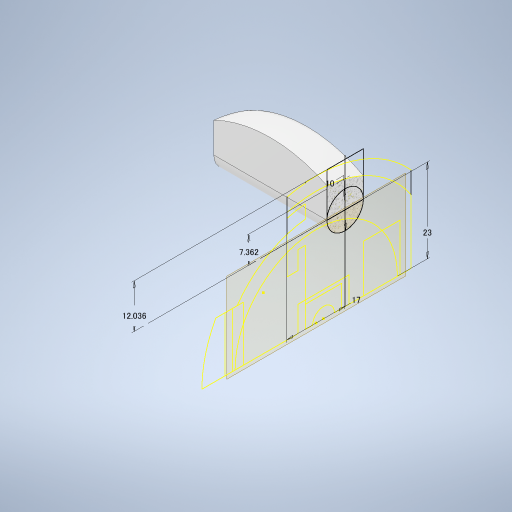
# Autodesk Inventor part: tail11-1
Saved by Autodesk Inventor 2023 (Build 270158000, 158)
## iProperties
Created: 2022-10-08
Part Number: tail11-1
Material: ABS プラスチック
Document SubType Name: Modeling
Designer: ellie
Density: 1.06 g/cm^3
Appearance: 積雪
Author: ellie
Autodesk Inventor part; units mm, degrees
sketch "スケッチ1" plane through (0, 0, 0) normal (0, 1, 0) x (-1, 0, 0)
  circle A0 centre (0, 0) radius 35
  line L0 (0, 0) -> (0, -35)
  line L1 (0, 0) -> (0, 35)
  dimension "d0" = 70
  constraints: 4 end point, 2 point on circle, 2 vertical, 1 centre point, 1 coincident
  measures "d0" diameter of A0
revolve "回転1" add sketch "スケッチ1" angle 180 about axis through (0, 0, 0) along (0, 0, 1) picked at (-2.5961, -23.0408) contours L1 L0 A0
sketch "スケッチ5" plane through (0, 0, 0) normal (0, -1, 0) x (1, 0, 0)
  line L0 (-20, -23) -> (20, -23)
  line L1 (20, -23) -> (20, -13)
  line L2 (20, -13) -> (-20, -13)
  line L3 (-20, -13) -> (-20, -23)
  line L4 (-20, -15) -> (-20, -13)
  line L5 (0, 25) -> (-17, 25)
  line L6 (-17, 25) -> (-17, 23)
  line L7 (-17, 23) -> (0, 23)
  line L8 (0, 23) -> (0, 25)
  line L9 (0, 20) -> (-20, 20)
  line L10 (-20, 20) -> (-20, 19)
  line L11 (-20, 19) -> (0, 19)
  line L12 (0, 19) -> (0, 20)
  line L13 (0, 13) -> (-21, 13)
  line L14 (-21, 13) -> (-21, 11)
  line L15 (-21, 11) -> (0, 11)
  line L16 (0, 11) -> (0, 13)
  line L17 (0, 5) -> (-23, 5)
  line L18 (-23, 5) -> (-23, 3)
  line L19 (-23, 3) -> (0, 3)
  line L20 (0, 3) -> (0, 5)
  circle A0 centre (0, 0) radius 35 projected
  circle A1 centre (0, 0) radius 35 projected
  line L21 (0, 35) -> (0, -35)
  line L22 (35, 0) -> (-35, 0)
  line L23 (-32, 3) -> (-23, 3)
  line L24 (-23, 3) -> (-23, -7)
  line L25 (-23, -7) -> (-32, -7)
  line L26 (-32, -7) -> (-32, 3)
  line L27 (-23, -8.0262) -> (-23, 3)
  line L28 (-27, 22.2711) -> (-27, -22.2711)
  line L29 (-15.5, 25) -> (0, 25)
  line L30 (0, 25) -> (0, 35)
  line L31 (0, 35) -> (-15.5, 35)
  line L32 (-15.5, 35) -> (-15.5, 25)
  line L33 (-15.5, 23) -> (0, 23)
  line L34 (0, 23) -> (0, 20)
  line L35 (0, 20) -> (-15.5, 20)
  line L36 (-15.5, 20) -> (-15.5, 23)
  line L37 (-19, 13) -> (0, 13)
  line L38 (0, 13) -> (0, 19)
  line L39 (0, 19) -> (-19, 19)
  line L40 (-19, 19) -> (-19, 13)
  line L41 (-19, 11) -> (0, 11)
  line L42 (0, 11) -> (0, 5)
  line L43 (0, 5) -> (-19, 5)
  line L44 (-19, 5) -> (-19, 11)
  line L45 (-23, -2) -> (-39.6865, -2)
  line L46 (-23, -2) -> (-7.8337, -2)
  line L47 (-8, 3) -> (-23, 3)
  line L48 (-23, 3) -> (-23, -7)
  line L49 (-23, -7) -> (-8, -7)
  line L50 (-8, -7) -> (-8, 3)
  line L51 (-8, 3) -> (-23, -7) construction
  line L52 (-23, 3) -> (-8, -7) construction
  line L53 (-23, 5) -> (-33, 5)
  line L54 (-33, 5) -> (-33, -9)
  line L55 (-33, -9) -> (-23, -9)
  line L56 (-23, -9) -> (-23, 5)
  line L57 (-23, 5) -> (-33, -9) construction
  line L58 (-33, 5) -> (-23, -9) construction
  line L59 (-8, 3) -> (-1, 3)
  line L60 (-1, 3) -> (-1, -7)
  line L61 (-1, -7) -> (-8, -7)
  line L62 (-8, -7) -> (-8, 3)
  line L63 (-8, 3) -> (-1, -7) construction
  line L64 (-1, 3) -> (-8, -7) construction
  line L65 (-23, 3) -> (-27, 3)
  line L66 (-23, -7) -> (-27, -7)
  line L67 (-23, 5) -> (-27, 5)
  line L68 (-23, -9) -> (-27, -9)
  line L69 (23.4307, -26) -> (-23.4307, -26)
  line L70 (-8, 3) -> (-6.8, 3)
  line L71 (-6.8, 3) -> (-6.8, -7)
  line L72 (-6.8, -7) -> (-8, -7)
  line L73 (-8, -7) -> (-8, 3)
  line L74 (-3, 5) -> (0, 5)
  line L75 (0, 20) -> (-4, 20)
  line L76 (-4, 19) -> (0, 19)
  line L77 (0, 19) -> (0, 20)
  line L78 (-6, 5) -> (-1, 5)
  line L79 (-1, 3) -> (-6, 3)
  point P0 (0, -23)
  point P1 (0, -13)
  point P2 (0, 24)
  point P3 (0, 19.5)
  point P4 (0, 12)
  point P5 (0, 4)
  point P6 (-20, -18)
  point P7 (-27, -0.5262)
  point P8 (-27, -7)
  point P9 (-15.5, 21.5)
  point P10 (-15.5, 31.3807)
  point P11 (0, 25)
  point P12 (0, 23)
  point P13 (0, 11)
  point P14 (0, 13)
  point P15 (-27, 0)
  point P16 (-32, 0)
  point P17 (-23, 0)
  point P18 (-15.5, -2)
  point P19 (-28, -2)
  point P20 (-4.5, -2)
  point P21 (-8, 3)
  point P22 (-27, 0.5)
  point P23 (-28, 0.4738)
  point P24 (-28, -11.5262)
  point P25 (-27, -11.5)
  point P26 (-23, -7)
  point P27 (-23, -7)
  point P28 (-23, -7)
  point P29 (-8, 0)
  point P30 (-1, 0)
  point P31 (0, 19)
  point P32 (0, 20)
  point P33 (-27, -9)
  point P34 (-27, 5)
  dimension "d12" = 40
  dimension "d13" = 10
  dimension "d23" = 17
  dimension "d24" = 2
  dimension "d27" = 20
  dimension "d28" = 1
  dimension "d30" = 21
  dimension "d31" = 2
  dimension "d33" = 2
  dimension "d88" = 0
  dimension "d89" = 0
  dimension "d90" = 12
  dimension "d92" = 20
  dimension "d93" = 10
  dimension "d97" = 9
  dimension "d98" = 10
  dimension "d113" = 27
  dimension "d122" = 15.5
  dimension "d123" = 35
  dimension "d124" = 3
  dimension "d125" = 15.5
  dimension "d126" = 6
  dimension "d127" = 6
  dimension "d128" = 19
  dimension "d129" = 19
  dimension "d147" = 10
  dimension "d149" = 8
  dimension "d151" = 15
  dimension "d161" = 14
  dimension "d162" = 10
  dimension "d164" = 10
  dimension "d165" = 7
  dimension "d170" = 26
  dimension "d175" = 1.2
  dimension "d207" = 0
  constraints: 158 end point, 31 parallel, 20 horizontal, 17 perpendicular, 16 point on line, 15 midpoint, 10 collinear, 1 vertical, 20 other
  measures "d12" distance of L2.end L1.end
  measures "d13" distance of L1.end L0.end
  measures "d23" distance of L7.end L6.end
  measures "d24" distance of L6.end L5.end
  measures "d27" distance of L11.end L10.end
  measures "d28" distance of L10.end L9.end
  measures "d30" distance of L15.end L14.end
  measures "d31" distance of L14.end L13.end
  measures "d33" distance of L18.end L17.end
  measures "d89" distance from line of point (0, 0) L22
  measures "d90" distance from line of L0 point (0, -35)
  measures "d92" distance of the line from the sketch origin of L3
  measures "d93" distance from line of L5 point (0, 35)
  measures "d97" distance of L24.end L25.end
  measures "d98" distance of L23.end L24.end
  measures "d113" distance of the line from the sketch origin of L28
  measures "d122" distance of the line from the sketch origin of L32
  measures "d123" distance between parallel lines of L31 L22
  measures "d124" distance of L33.end L34.end
  measures "d126" distance of L38.end L37.end
  measures "d127" distance of L41.end L42.end
  measures "d128" distance of the line from the sketch origin of L44
  measures "d129" distance of the line from the sketch origin of L40
  measures "d147" distance of L48.end L47.end
  measures "d149" distance of the line from the sketch origin of L50
  measures "d151" distance between parallel lines of L50 L24
  measures "d161" distance between parallel lines of L55 L53
  measures "d162" distance between parallel lines of L48 L54
  measures "d164" distance between parallel lines of L61 L59
  measures "d165" distance between parallel lines of L50 L60
  measures "d170" distance between parallel lines of L69 L22
  measures "d175" distance of L71.end L72.end
  measures "d207" distance between parallel lines of L47 L19
extrude "GNSボード" cut sketch "スケッチ5" against normal blind 16 contours L8 L7 L6 L5
extrude "GNSボード止めるよう" cut sketch "スケッチ5" against normal blind 15 contours L21 L5 L32 A0 | L21 L9 L36 L7
extrude "アルミ板１" cut sketch "スケッチ5" against normal blind 20 contours L11 L10 L9 L12
extrude "メイン基板" cut sketch "スケッチ5" against normal blind 21 contours L15 L14 L13 L16
extrude "メイン止めるよう" cut sketch "スケッチ5" against normal blind 15 contours L17 L44 L15 L21 | L13 L40 L11 L21
extrude "アルミ板２" cut sketch "スケッチ5" against normal blind 20 contours L19 L18 L17 L20
extrude "電池ボックス入れ" cut sketch "スケッチ5" against normal blind 13 contours L3 L2 L21 L0 | L21 L2 L1 L0
extrude "side ut" cut sketch "スケッチ5" against normal blind 100 contours A0 L45 L54 L55 L28 | A0 L22 L54 L45 | L55 L54 L45 L26 L25 L28 | A0 L28 L53 L54 L22 | L54 L22 L26 L45 | L25 L26 L45 L28 | L54 L53 L28 L23 L26 L22 | L26 L22 L28 L45 | L22 L26 L23 L28
extrude "motor case" add sketch "スケッチ5" against normal blind 7 contours L55 L54 L45 L26 L25 L28 | L28 L25 L27 L56 L55 | L50 L46 L24 L22 | L22 L24 L19 L50 | L54 L22 L26 L45 | L28 L45 L24 L25 | L25 L26 L45 L28 | L24 L45 L28 L22 | L22 L28 L23 L24 | L50 L49 L24 L46 | L54 L53 L28 L23 L26 L22 | L26 L22 L28 L45 | L53 L18 L23 L28 | L22 L26 L23 L28
extrude "bottom cut" cut sketch "スケッチ5" against normal blind 90 contours L69 A0 L21 | L21 A0 L69
extrude "motor" cut sketch "スケッチ5" against normal blind 6 contours L60 L61 L71 L22 | L22 L71 L19 L60 | L71 L61 L50 L22 | L22 L50 L19 L71 | L50 L46 L24 L22 | L22 L24 L19 L50 | L28 L45 L24 L25 | L25 L26 L45 L28 | L24 L45 L28 L22 | L22 L28 L23 L24 | L50 L49 L24 L46 | L26 L22 L28 L45 | L22 L26 L23 L28
extrude "motor block" add sketch "スケッチ5" against normal blind 10 contours L71 L61 L50 L22 | L22 L50 L19 L71
sketch "スケッチ27" plane through (-33, 0, -9) normal (-1, 0, 0) x (0, 0, 1)
  line L0 (14, 0) -> (0, 0) projected
  circle A0 centre (7, 0) radius 3
  point P0 (9, 0)
  dimension "d198" = 6
  constraints: 1 centre point, 1 midpoint
  measures "d198" diameter of A0
extrude "moter shaft" cut sketch "スケッチ27" against normal blind 27
mirror "ミラー13" about plane through (0, 0, 0) normal (1, 0, 0) of "メイン止めるよう", "メイン基板", "アルミ板１", "GNSボード止めるよう", "GNSボード", "アルミ板２", "motor", "motor case", "moter shaft", "電池ボックス入れ", "side ut", "motor block"
ref_plane "作業平面5" through (-17, 17.5, 23) normal (0, -1, 0) x (1, 0, 0)
ref_plane "作業平面6" through (20, 13, -13) normal (0, 0, -1) x (1, 0, 0)
ref_plane "作業平面7" through (27, 11.5, 5) normal (0, -1, 0) x (1, 0, 0)
sketch "スケッチ41" plane through (-17, 0, 23) normal (0, -1, 0) x (1, 0, 0)
  line L0 (-16, -22) -> (-15, -22) projected
  line L1 (-15, -22) -> (-15, -20) projected
  line L2 (-15, -20) -> (-6, -20) projected
  line L3 (-6, -20) -> (-6, -18) projected
  line L4 (-6, -18) -> (-2, -18) projected
  line L5 (-2, -18) -> (-2, -12) projected
  line L6 (-2, -12) -> (-4, -12) projected
  line L7 (-4, -12) -> (-4, -10) projected
  line L8 (-4, -10) -> (-2, -10) projected
  line L9 (-2, -10) -> (-2, -4) projected
  line L10 (-2, -4) -> (-3, -4) projected
  line L11 (-3, -4) -> (-3, -3) projected
  line L12 (-3, -3) -> (1.5, -3) projected
  line L13 (1.5, -3) -> (1.5, 0) projected
  line L14 (1.5, 0) -> (0, 0) projected
  line L15 (0, 0) -> (0, 2) projected
  line L16 (0, 2) -> (1.5, 2) projected
  line L17 (1.5, 2) -> (1.5, 8.3807) projected
  arc A0 (1.5, 8.3807) -> (-10, -0.7289) centre (17, -23) ccw projected
  line L18 (-10, -0.7289) -> (-10, -18) projected
  line L19 (-10, -18) -> (-16, -18) projected
  line L20 (-16, -18) -> (-16, -22) projected
  line L21 (-2, -18) -> (-2, -12) projected
  line L22 (-4, -10) -> (-4, -12) projected
  line L23 (0, 2) -> (0, 0) projected
  circle A1 centre (-4, 0.5) radius 2.4
  dimension "d252" = 4.8
  dimension "d253" = 4
  dimension "d254" = 3.5
  constraints: 1 centre point
  measures "d252" diameter of A1
  measures "d253" distance from line of A1.centre L15
  measures "d254" distance from line of A1.centre L12
extrude "top lock 10mm" cut sketch "スケッチ41" against normal blind 3 contours A1
mirror "ミラー15" about plane through (0, 0, 0) normal (1, 0, 0) of "top lock 10mm"
sketch "スケッチ42" plane through (-33, 0, -9) normal (0, -1, 0) x (1, 0, 0)
  circle A0 centre (9.5, -8) radius 2.4
  line L0 (13, -14) -> (13, -4) projected
  line L1 (32, 2) -> (1, 2) projected
  point P0 (33, 9)
  point P1 (10, 2)
  dimension "d257" = 3.5
  dimension "d258" = 4.8
  dimension "d259" = 10
  constraints: 1 centre point
  measures "d257" distance from line of A0.centre L0
  measures "d258" diameter of A0
  measures "d259" distance from line of A0.centre L1
extrude "bottom lock" cut sketch "スケッチ42" against normal blind 3
mirror "ミラー16" about plane through (0, 0, 0) normal (1, 0, 0) of "bottom lock"
ref_plane "作業平面8" through (-17, 15, 23) normal (0, -1, 0) x (1, 0, 0)
sketch "スケッチ45" plane through (-17, 15, 23) normal (0, -1, 0) x (1, 0, 0)
  circle A0 centre (-4, 0.5) radius 2.4 projected
  line L0 (-16, -22) -> (-15, -22) projected
  line L1 (-15, -22) -> (-15, -20) projected
  line L2 (-15, -20) -> (-6, -20) projected
  line L3 (-6, -20) -> (-6, -18) projected
  line L4 (-6, -18) -> (-2, -18) projected
  line L5 (-2, -18) -> (-2, -12) projected
  line L6 (-2, -12) -> (-4, -12) projected
  line L7 (-4, -12) -> (-4, -10) projected
  line L8 (-4, -10) -> (-2, -10) projected
  line L9 (-2, -10) -> (-2, -4) projected
  line L10 (-2, -4) -> (-3, -4) projected
  line L11 (-3, -4) -> (-3, -3) projected
  line L12 (-3, -3) -> (1.5, -3) projected
  line L13 (1.5, -3) -> (1.5, 0) projected
  line L14 (1.5, 0) -> (0, 0) projected
  line L15 (0, 0) -> (0, 2) projected
  line L16 (0, 2) -> (1.5, 2) projected
  line L17 (1.5, 2) -> (1.5, 8.3807) projected
  arc A1 (1.5, 8.3807) -> (-10, -0.7289) centre (17, -23) ccw projected
  line L18 (-10, -0.7289) -> (-10, -18) projected
  line L19 (-10, -18) -> (-16, -18) projected
  line L20 (-16, -18) -> (-16, -22) projected
  arc A2 (32.5, 4.5636) -> (1.5, 4.5636) centre (17, -23) ccw projected
  line L21 (1.5, 2) -> (1.5, 4.5636) projected
  line L22 (32.5, 2) -> (1.5, 2) projected
  line L23 (32.5, 2) -> (32.5, 4.5636) projected
  circle A3 centre (38, 0.5) radius 2.4 projected
  line L24 (49, -22) -> (50, -22) projected
  line L25 (50, -18) -> (50, -22) projected
  line L26 (44, -18) -> (50, -18) projected
  line L27 (44, -18) -> (44, -0.7289) projected
  arc A4 (44, -0.7289) -> (32.5, 8.3807) centre (17, -23) ccw projected
  line L28 (32.5, 8.3807) -> (32.5, 2) projected
  line L29 (32.5, 2) -> (34, 2) projected
  line L30 (34, 2) -> (34, 0) projected
  line L31 (34, 0) -> (32.5, 0) projected
  line L32 (32.5, 0) -> (32.5, -3) projected
  line L33 (32.5, -3) -> (37, -3) projected
  line L34 (37, -3) -> (37, -4) projected
  line L35 (37, -4) -> (36, -4) projected
  line L36 (36, -4) -> (36, -10) projected
  line L37 (36, -10) -> (38, -10) projected
  line L38 (38, -10) -> (38, -12) projected
  line L39 (38, -12) -> (36, -12) projected
  line L40 (36, -12) -> (36, -18) projected
  line L41 (36, -18) -> (40, -18) projected
  line L42 (40, -18) -> (40, -20) projected
  line L43 (40, -20) -> (49, -20) projected
  line L44 (49, -20) -> (49, -22) projected
  circle A5 centre (38, 0.5) radius 2.4 projected
  circle A6 centre (-4, 0.5) radius 2.4 projected
  line L45 (34, 0) -> (0, 0) projected
  line L46 (34, 0) -> (34, 2) projected
  line L47 (34, 2) -> (0, 2) projected
  line L48 (0, 0) -> (0, 2) projected
  line L49 (32.5, -3) -> (1.5, -3) projected
  line L50 (32.5, -3) -> (32.5, 0) projected
  line L51 (1.5, 0) -> (32.5, 0) projected
  line L52 (1.5, -3) -> (1.5, 0) projected
  line L53 (-2, -4) -> (36, -4) projected
  circle A7 centre (38, 0.5) radius 2.4 projected
  line L54 (36, -10) -> (-2, -10) projected
  line L55 (36, -10) -> (36, -4) projected
  line L56 (-2, -4) -> (36, -4) projected
  line L57 (-2, -10) -> (-2, -4) projected
  line L58 (-2, -12) -> (36, -12) projected
  line L59 (36, -18) -> (-2, -18) projected
  line L60 (36, -18) -> (36, -12) projected
  line L61 (-2, -12) -> (36, -12) projected
  line L62 (-2, -18) -> (-2, -12) projected
  line L63 (40, -20) -> (-6, -20) projected
  line L64 (40, -20) -> (40, -18) projected
  line L65 (40, -18) -> (-6, -18) projected
  line L66 (-6, -20) -> (-6, -18) projected
  line L67 (9, -30) -> (9, -20) projected
  line L68 (-6, -20) -> (9, -20) projected
  line L69 (-15, -20) -> (-6, -20) projected
  line L70 (-15, -30) -> (-15, -20) projected
  line L71 (16, -30) -> (10.2, -30) projected
  circle A8 centre (40.5, -40) radius 2.4 projected
  circle A9 centre (-6.5, -40) radius 2.4 projected
  line L72 (25, -28) -> (23.8, -28) projected
  line L73 (23.8, -30) -> (23.8, -28) projected
  line L74 (18, -30) -> (18, -20) projected
  line L75 (18, -20) -> (16, -20) projected
  line L76 (16, -20) -> (16, -30) projected
  line L77 (10.2, -30) -> (10.2, -28) projected
  line L78 (10.2, -28) -> (9, -28) projected
  line L79 (9, -20) -> (9, -22) projected
  line L80 (-6, -20) -> (-6, -18) projected
  line L81 (16, -30) -> (10.2, -30) projected
  line L82 (-15, -30) -> (-15, -28) projected
  line L83 (-15, -28) -> (-16, -28) projected
  line L84 (-16, -28) -> (-16, -32) projected
  line L85 (-16, -32) -> (-10, -32) projected
  line L86 (-10, -32) -> (-10, -45.2711) projected
  arc A10 (-10, -45.2711) -> (-6.4307, -49) centre (17, -23) ccw projected
  line L87 (-6.4307, -49) -> (40.4307, -49) projected
  arc A11 (40.4307, -49) -> (44, -45.2711) centre (17, -23) ccw projected
  line L88 (44, -45.2711) -> (44, -32) projected
  line L89 (50, -32) -> (44, -32) projected
  line L90 (50, -28) -> (50, -32) projected
  line L91 (50, -28) -> (49, -28) projected
  line L92 (49, -28) -> (49, -30) projected
  line L93 (23.8, -30) -> (18, -30) projected
  line L94 (40, -18) -> (40, -20) projected
  line L95 (25, -20) -> (25, -22) projected
  line L96 (-3, -36) -> (37, -36) projected
  line L97 (37, -36) -> (37, -46) projected
  line L98 (37, -46) -> (-3, -46) projected
  line L99 (-3, -46) -> (-3, -36) projected
  line L100 (-6, -15) -> (40, -15)
  line L101 (40, -15) -> (40, 8.6228)
  line L102 (40, 8.6228) -> (-6, 8.6228)
  line L103 (-6, 8.6228) -> (-6, -15)
  line L104 (10.2, -20) -> (10.2, -30) projected
  line L105 (16, -20) -> (16, -30) projected
  line L106 (10.2, -20) -> (16, -20) projected
  line L107 (9, -30) -> (-15, -30) projected
  line L108 (-16, -22) -> (-15, -22) projected
  line L109 (-15, -22) -> (-15, -20) projected
  line L110 (-15, -20) -> (-6, -20) projected
  line L111 (-6, -18) -> (-2, -18) projected
  line L112 (-2, -18) -> (-2, -12) projected
  line L113 (-2, -12) -> (-4, -12) projected
  line L114 (-4, -12) -> (-4, -10) projected
  line L115 (-4, -10) -> (-2, -10) projected
  line L116 (-2, -10) -> (-2, -4) projected
  line L117 (-2, -4) -> (-3, -4) projected
  line L118 (-3, -4) -> (-3, -3) projected
  line L119 (-3, -3) -> (1.5, -3) projected
  line L120 (1.5, -3) -> (1.5, 0) projected
  line L121 (1.5, 0) -> (0, 0) projected
  line L122 (0, 0) -> (0, 2) projected
  line L123 (0, 2) -> (1.5, 2) projected
  line L124 (1.5, 2) -> (1.5, 8.3807) projected
  arc A12 (1.5, 8.3807) -> (-10, -0.7289) centre (17, -23) ccw projected
  line L125 (-10, -0.7289) -> (-10, -18) projected
  line L126 (-10, -18) -> (-16, -18) projected
  line L127 (-16, -18) -> (-16, -22) projected
  line L128 (9, -22) -> (10.2, -22) projected
  line L129 (10.2, -22) -> (10.2, -20) projected
  line L130 (10.2, -20) -> (9, -20) projected
  line L131 (9, -28) -> (9, -30) projected
  line L132 (9, -30) -> (-15, -30) projected
  line L133 (49, -30) -> (25, -30) projected
  line L134 (25, -28) -> (25, -30) projected
  line L135 (23.8, -22) -> (25, -22) projected
  line L136 (23.8, -20) -> (25, -20) projected
  line L137 (23.8, -22) -> (23.8, -20) projected
  line L138 (49, -22) -> (50, -22) projected
  line L139 (50, -18) -> (50, -22) projected
  line L140 (44, -18) -> (50, -18) projected
  line L141 (44, -18) -> (44, -0.7289) projected
  arc A13 (44, -0.7289) -> (32.5, 8.3807) centre (17, -23) ccw projected
  line L142 (32.5, 8.3807) -> (32.5, 2) projected
  line L143 (32.5, 2) -> (34, 2) projected
  line L144 (34, 2) -> (34, 0) projected
  line L145 (34, 0) -> (32.5, 0) projected
  line L146 (32.5, 0) -> (32.5, -3) projected
  line L147 (32.5, -3) -> (37, -3) projected
  line L148 (37, -3) -> (37, -4) projected
  line L149 (37, -4) -> (36, -4) projected
  line L150 (36, -4) -> (36, -10) projected
  line L151 (36, -10) -> (38, -10) projected
  line L152 (38, -10) -> (38, -12) projected
  line L153 (38, -12) -> (36, -12) projected
  line L154 (36, -12) -> (36, -18) projected
  line L155 (36, -18) -> (40, -18) projected
  line L156 (40, -20) -> (49, -20) projected
  line L157 (49, -20) -> (49, -22) projected
  dimension "d269" = 3
  constraints: 8 end point, 2 collinear, 2 parallel, 1 horizontal, 1 perpendicular, 1 tangent
  measures "d269" distance between parallel lines of L100 L65
extrude "back cut" cut sketch "スケッチ45" against normal blind 20 contours A0 L103 | A0 L103 A1 L17 L16 L15 L14 L13 L12 L11 L10 L9 L8 L7 L6 L5 L100 | L103 L102 A2 L17 A1 | L5 L58 L40 L100 | A2 L23 L22 L17 | L102 L101 A4 L28 A2 | L6 L7 L8 L54 L37 L38 L39 L58 | L40 L39 L38 L37 L36 L35 L34 L33 L32 L31 L30 L29 L23 L28 A4 L101 A3 L100 | L22 L29 L30 L31 L45 L14 L15 L16 | A3 L101 | L9 L53 L36 L54 | L45 L32 L49 L13 | L10 L11 L12 L49 L33 L34 L35 L53 picked at (-4.4805, 1.0136) picked at (38.5393, 0.5971)
sketch "スケッチ52" plane through (20, 0, -13) normal (0, 0, -1) x (-1, 0, 0)
  line L0 (40, 0) -> (0, 0) projected
  line L1 (40, 0) -> (40, 13) projected
  line L2 (40, 13) -> (0, 13) projected
  line L3 (0, 0) -> (0, 13) projected
  line L4 (28, 0) -> (28, 6) projected
  line L5 (28, 6) -> (52, 6) projected
  line L6 (52, 0) -> (52, 6) projected
  line L7 (28, 0) -> (52, 0) projected
  line L8 (26.8, 6) -> (26.8, 0) projected
  line L9 (21, 0) -> (26.8, 0) projected
  line L10 (21, 0) -> (21, 6) projected
  line L11 (21, 6) -> (26.8, 6) projected
  line L12 (13.2, 0) -> (13.2, 6) projected
  line L13 (19, 6) -> (13.2, 6) projected
  line L14 (19, 0) -> (19, 6) projected
  line L15 (13.2, 0) -> (19, 0) projected
  line L16 (12, 6) -> (12, 0) projected
  line L17 (-12, 0) -> (12, 0) projected
  line L18 (-12, 0) -> (-12, 6) projected
  line L19 (12, 6) -> (-12, 6) projected
  line L20 (27, 10) -> (37, 10)
  line L21 (37, 10) -> (37, 16)
  line L22 (37, 16) -> (27, 16)
  line L23 (27, 16) -> (27, 10)
  point P0 (20, 0)
  dimension "d293" = 3
  dimension "d294" = 10
  dimension "d295" = 4
  constraints: 8 end point, 2 parallel, 1 horizontal, 1 perpendicular, 1 other
  measures "d293" distance between parallel lines of L1 L21
  measures "d294" distance between parallel lines of L21 L23
  measures "d295" distance between parallel lines of L20 L5
extrude "押し出し54" cut sketch "スケッチ52" against normal up to surface (18 mm away) contours L21 L20 L23 L2 | L2 L23 L22 L21
sketch "スケッチ53" plane through (0, 13, 0) normal (0, -1, 0) x (1, 0, 0)
  line L0 (-7, -13) -> (-7, 3) projected
  line L1 (-17, -13) -> (-7, -13) projected
  line L2 (-17, -13) -> (-17, 3) projected
  line L3 (-17, -13) -> (-17, 3) projected
  line L4 (-17, -13) -> (-17, 3) projected
  line L5 (-23, 8) -> (23, 8) projected
  line L6 (23, 8) -> (23, 21.7025) projected
  arc A0 (23, 21.7025) -> (15.5, 27.5636) centre (0, 0) ccw projected
  line L7 (15.5, 27.5636) -> (15.5, 31.3807) projected
  arc A1 (27, 22.2711) -> (15.5, 31.3807) centre (0, 0) ccw projected
  line L8 (27, 22.2711) -> (27, -22.2711) projected
  arc A2 (23.4307, -26) -> (27, -22.2711) centre (0, 0) ccw projected
  line L9 (23.4307, -26) -> (-23.4307, -26) projected
  arc A3 (-27, -22.2711) -> (-23.4307, -26) centre (0, 0) ccw projected
  line L10 (-27, -22.2711) -> (-27, 22.2711) projected
  arc A4 (-15.5, 31.3807) -> (-27, 22.2711) centre (0, 0) ccw projected
  line L11 (-15.5, 31.3807) -> (-15.5, 27.5636) projected
  arc A5 (-15.5, 27.5636) -> (-23, 21.7025) centre (0, 0) ccw projected
  line L12 (-23, 21.7025) -> (-23, 8) projected
  line L13 (-17, -13) -> (-7, -13)
  line L14 (-7, -13) -> (-7, -19)
  line L15 (-7, -19) -> (-17, -19)
  line L16 (-17, -19) -> (-17, -13)
  dimension "d298" = 6
  constraints: 8 end point, 3 collinear, 2 parallel, 1 horizontal, 1 perpendicular
  measures "d298" distance between parallel lines of L15 L1
extrude "押し出し55" cut sketch "スケッチ53" against normal up to surface (3 mm away) contours L1 L14 L15 L16
sketch "スケッチ54" plane through (-23, 15, 8) normal (0, 0, 1) x (1, 0, 0)
  line L0 (42, 0) -> (46, 0) projected
  line L1 (46, 0) -> (41, 0)
  line L2 (41, 0) -> (41, 20)
  line L3 (41, 20) -> (46, 20)
  line L4 (46, 20) -> (46, 0)
  line L5 (0, 0) -> (4, 0) projected
  line L6 (0, 0) -> (5, 0)
  line L7 (5, 0) -> (5, 20)
  line L8 (5, 20) -> (0, 20)
  line L9 (0, 20) -> (0, 0)
  line L10 (23, -15) -> (23, 20)
  arc A0 (50, 7.2711) -> (-4, 7.2711) centre (23, -15) ccw projected
  line L11 (25.5, 0) -> (20.5, 0)
  line L12 (20.5, 0) -> (20.5, 20)
  line L13 (20.5, 20) -> (25.5, 20)
  line L14 (25.5, 20) -> (25.5, 0)
  line L15 (42, 0) -> (4, 0) projected
  arc A1 (46, 10.1396) -> (0, 10.1396) centre (23, -15) ccw projected
  line L16 (0, 0) -> (0, 10.1396) projected
  line L17 (0, 0) -> (4, 0) projected
  line L18 (42, 0) -> (4, 0) projected
  line L19 (42, 0) -> (46, 0) projected
  line L20 (46, 0) -> (46, 10.1396) projected
  line L21 (46, 0) -> (38.5, 0) projected
  line L22 (38.5, 0) -> (38.5, -15) projected
  line L23 (38.5, -15) -> (50, -15) projected
  line L24 (50, -15) -> (50, -15) projected
  line L25 (50, -15) -> (46.4307, -15) projected
  arc A2 (46.4307, -15) -> (-0.4307, -15) centre (23, -15) ccw projected
  line L26 (-0.4307, -15) -> (-4, -15) projected
  line L27 (-4, -15) -> (-4, -15) projected
  line L28 (-4, -15) -> (7.5, -15) projected
  line L29 (7.5, -15) -> (7.5, 0) projected
  line L30 (7.5, 0) -> (0, 0) projected
  line L31 (0, 0) -> (0, 10.1396) projected
  arc A3 (46, 10.1396) -> (0, 10.1396) centre (23, -15) ccw projected
  line L32 (46, 10.1396) -> (46, 0) projected
  point P0 (20.5, 0)
  point P1 (20.5, 19.9106)
  point P2 (5, 15.0167)
  point P3 (41, 15.0167)
  point P4 (25.5, 19.9106)
  point P5 (25.5, 0)
  point P6 (41, 13.931)
  point P7 (25.5, 18.9816)
  point P8 (20.5, 18.9816)
  point P9 (5, 13.931)
  point P10 (0, 10.1396)
  point P11 (46, 11.3818)
  point P12 (0, 11.3818)
  dimension "d301" = 5
  dimension "d302" = 5
  dimension "d303" = 2.5
  dimension "d304" = 5
  constraints: 26 end point, 6 parallel, 3 horizontal, 3 perpendicular, 3 tangent, 1 collinear, 1 point on circle, 1 vertical
  measures "d301" distance of L2.end L3.end
  measures "d302" distance of L8.end L7.end
  measures "d303" distance between parallel lines of L14 L10
  measures "d304" distance between parallel lines of L14 L12
extrude "押し出し56" cut sketch "スケッチ54" against normal up to surface (5 mm away) contours L1 L2 A1 L4 L0 | A1 L2 A0 L4 | A2 L10 A1 L14 | L14 L11 L10 A2 | A1 L10 A0 L14 | A2 L12 A1 L10 | L10 L11 L12 A2 | A0 L13 L14 | A1 L12 A0 L10 | A0 L12 L13 | L6 L5 L9 A1 L7 | A1 L9 A0 L7
ref_plane "作業平面9" through (15.5, 0, -9) normal (1, 0, 0) x (0, 0, -1)
sketch "スケッチ55" plane through (15.5, 0, -9) normal (1, 0, 0) x (0, 0, -1)
  arc A0 (-12, 29.8664) -> (-17, 28.931) centre (-9, 0) ccw projected
  line L0 (-12, 29.8664) -> (-12, 26.2107) projected
  arc A1 (-12, 26.2107) -> (-30.7025, 15) centre (-9, 0) ccw projected
  line L1 (-30.7025, 15) -> (-36.5636, 15) projected
  arc A2 (-36.5636, 15) -> (-40.3807, 0) centre (-9, 0) ccw projected
  line L2 (-40.3807, 0) -> (-31.2711, 0) projected
  arc A3 (13.2711, 0) -> (-31.2711, 0) centre (-9, 0) ccw projected
  line L3 (13.2711, 0) -> (17, 0) projected
  line L4 (17, 0) -> (17, 0) projected
  line L5 (17, 0) -> (13.2711, 0) projected
  arc A4 (13.2711, 0) -> (-31.2711, 0) centre (-9, 0) ccw projected
  line L6 (-31.2711, 0) -> (-40.3807, 0) projected
  arc A5 (-36.5636, 15) -> (-40.3807, 0) centre (-9, 0) ccw projected
  line L7 (-36.5636, 15) -> (-30.7025, 15) projected
  arc A6 (-12, 26.2107) -> (-30.7025, 15) centre (-9, 0) ccw projected
  line L8 (-12, 26.2107) -> (-12, 29.8664) projected
  arc A7 (-12, 29.8664) -> (-17, 28.931) centre (-9, 0) ccw projected
  line L9 (-17, 28.931) -> (-17, 33.9816) projected
  arc A8 (-12, 34.7815) -> (-17, 33.9816) centre (-9, 0) ccw projected
  line L10 (-12, 34.7815) -> (-12, 34.7815) projected
  arc A9 (-12, 34.7815) -> (-17, 33.9816) centre (-9, 0) ccw projected
  line L11 (-17, 33.9816) -> (-17, 28.931) projected
  line L12 (-14, 7) -> (-14, 0) projected
  line L13 (-31.2711, 0) -> (-14, 0) projected
  arc A10 (13.2711, 0) -> (-31.2711, 0) centre (-9, 0) ccw projected
  line L14 (0, 0) -> (13.2711, 0) projected
  line L15 (0, 0) -> (0, 7) projected
  line L16 (0, 7) -> (-14, 7) projected
  arc A11 (-4, 0) -> (-10, 0) centre (-7, 0) ccw projected
  line L17 (-10, 0) -> (-12, 0) projected
  line L18 (-12, 0) -> (-12, 6) projected
  line L19 (-2, 6) -> (-12, 6) projected
  line L20 (-2, 0) -> (-2, 6) projected
  line L21 (-2, 0) -> (-4, 0) projected
  line L22 (17, 0) -> (17, 0) projected
  circle A12 centre (-1.0682, 23) radius 5
  line L23 (-1.0682, 23) -> (-1.0682, 0)
  line L24 (-1.0682, 0) -> (-1.0682, 23)
  line L25 (-1.0682, 0) -> (-1.0682, 35.956)
  line L26 (-4, 0) -> (0, 0) projected
  line L27 (3.9317, 22.964) -> (-6.0682, 22.964)
  arc A13 (17, 23.4307) -> (-12, 34.8712) centre (-9, 0) ccw projected
  line L28 (-6.0682, 22.964) -> (3.9318, 22.964)
  line L29 (3.9318, 22.964) -> (3.9318, 35)
  line L30 (3.9318, 35) -> (-6.0682, 35)
  line L31 (-6.0682, 35) -> (-6.0682, 22.964)
  arc A14 (-36.5636, 15) -> (-40.3807, 0) centre (-9, 0) ccw projected
  line L32 (-36.5636, 15) -> (-34, 15) projected
  line L33 (-34, 15) -> (-34, 0) projected
  line L34 (-34, 0) -> (-40.3807, 0) projected
  line L35 (-32, 15) -> (-29, 15) projected
  line L36 (-29, 15) -> (-29, 0) projected
  line L37 (-29, 0) -> (-32, 0) projected
  line L38 (-32, 0) -> (-32, 15) projected
  line L39 (17, 0) -> (14, 0) projected
  line L40 (14, 0) -> (14, 13) projected
  line L41 (14, 13) -> (4, 13) projected
  line L42 (4, 13) -> (4, 0) projected
  line L43 (4, 0) -> (-2, 0) projected
  line L44 (-2, 0) -> (-2, 6) projected
  line L45 (-2, 6) -> (-12, 6) projected
  line L46 (-12, 6) -> (-12, 20) projected
  line L47 (-12, 20) -> (-14, 20) projected
  line L48 (-14, 20) -> (-14, 15) projected
  line L49 (-14, 15) -> (-17, 15) projected
  line L50 (-17, 15) -> (-17, 30.3439) projected
  arc A15 (17, 17.5713) -> (-17, 30.3439) centre (-9, 0) ccw projected
  line L51 (17, 17.5713) -> (17, 0) projected
  line L52 (17, 17.5713) -> (17, 23.4307)
  line L53 (-17, 33.9816) -> (-17, 25.1396)
  line L54 (-12, 34.8712) -> (-12, 34.7815)
  point P0 (-1.0682, 30.3617)
  point P1 (3.9318, 23)
  point P2 (-17, 30.3617)
  point P3 (3.9317, 22.964)
  point P4 (-12, 7)
  point P5 (3.9318, 28.5923)
  point P6 (3.9317, 22.964)
  point P7 (-6.068, 22.964)
  point P8 (-6.0682, 31.2435)
  point P9 (13.2711, 0)
  point P10 (-17, 25.1396)
  point P11 (3.9318, 32.5233)
  point P12 (-12, 34.7815)
  point P13 (-6.0682, 34.877)
  dimension "d313" = 10
  dimension "d311" = 17
  dimension "d312" = 23
  dimension "d324" = 7.3617
  dimension "d329" = 12.036
  constraints: 22 end point, 5 vertical, 3 equal length, 3 point on line, 2 horizontal, 2 perpendicular, 1 coincident, 1 point on circle, 1 tangent, 3 other
  measures "d311" distance of L23.start L11.end
  measures "d312" distance from line of L23.start L14
  measures "d324" distance of L23.start point (-1.068, 30.362)
  measures "d329" distance of L30.end L27.end
extrude "押し出し63" cut sketch "スケッチ55" against normal up to surface (31 mm away) contours L0 A1 L50 A0 | A0 L9 A15 L31 A12 A3 L50 A1 L0 | L9 A8 L54 A13 L31 A15 | L50 A3 L36 L35 A1 | L35 L36 A3 L2 L38 L1 | L50 L49 L48 L47 L46 L16 L12 L13 L36 A3 | A3 A12 L23 L16 L46 L47 L48 L49 L50 | L38 L2 L33 L1 | L36 L13 A3 | A15 L51 L3 L40 L41 A3 A12 L29 | L29 A13 L52 A15 | L33 L2 A2 L1 | A12 A3 L41 L42 L14 L15 L16 L23 | L23 L26 L20 L19 L46 L16 | L16 L15 L26 L23 | L41 L40 L3 A3 | A3 L14 L42 L41 | L19 L20 L21 A11 L17 L18
sketch "スケッチ58" plane through (1, 0, -2) normal (1, 0, 0) x (0, 0, -1)
  point P0 (-2, 0)
extrude "押し出し64" cut sketch "スケッチ55" against normal blind 1000 contours L0 A1 L50 A0 | A0 L9 A15 L31 A12 A3 L50 A1 L0 | L50 A3 L36 L35 A1 | L35 L36 A3 L2 L38 L1 | L50 L49 L48 L47 L46 L16 L12 L13 L36 A3 | A3 A12 L23 L16 L46 L47 L48 L49 L50 | L38 L2 L33 L1 | L36 L13 A3 | A15 L51 L3 L40 L41 A3 A12 L29 | L33 L2 A2 L1 | A12 A3 L41 L42 L14 L15 L16 L23 | L23 L26 L20 L19 L46 L16 | L16 L15 L26 L23 | L41 L40 L3 A3 | A3 L14 L42 L41 | L19 L20 L21 A11 L17 L18
sketch "スケッチ59" plane through (-33, 0, 5) normal (-1, 0, 0) x (0, 0, 1)
  line L0 (-2, 7) -> (-2, 0) projected
  line L1 (-2, 0) -> (0, 0) projected
  line L2 (-2, 0) -> (-2, 7) projected
  line L3 (0, 0) -> (-2, 0)
  line L4 (-2, 0) -> (-2, 7)
  line L5 (-2, 7) -> (0, 7)
  line L6 (0, 7) -> (0, 0)
  line L7 (-10, 0) -> (-4, 0) projected
  circle A0 centre (-7, 0) radius 3
  line L8 (0, 0) -> (-10, 0)
  point P0 (-5, 0)
  dimension "d339" = 6
  constraints: 10 end point, 2 horizontal, 2 parallel, 1 centre point, 1 midpoint, 1 perpendicular
  measures "d339" diameter of A0
extrude "押し出し65" cut sketch "スケッチ59" against normal blind 1000
sketch "スケッチ60" plane through (-27, 23, -7.9318) normal (-1, 0, 0) x (0, 0.3260206, 0.9453627)
  arc A0 (-4.3388, -2.485) -> (4.3388, -2.485) centre (0, 0) ccw projected
  arc A1 (4.3388, -2.485) -> (-4.3388, -2.485) centre (0, -24.3293) ccw projected
  line L0 (4.7151, -1.6642) -> (7.4144, 6.163) projected
  arc A2 (17.4556, 1.7485) -> (7.4144, 6.163) centre (0, -24.3293) ccw projected
  line L1 (17.4556, 1.7485) -> (16.995, 0.4128) projected
  arc A3 (16.995, 0.4128) -> (12.5731, 2.9272) centre (0, -24.3293) ccw projected
  line L2 (12.5731, 2.9272) -> (11.3813, -0.5287) projected
  arc A4 (25.4071, -17.2243) -> (11.3813, -0.5287) centre (0, -24.3293) ccw projected
  line L3 (25.4071, -17.2243) -> (30.9479, -19.1351) projected
  arc A5 (29.6662, -34.5601) -> (30.9479, -19.1351) centre (0, -24.3293) ccw projected
  line L4 (29.6662, -34.5601) -> (21.0542, -31.5901) projected
  arc A6 (21.0542, -31.5901) -> (-21.0542, -17.0685) centre (0, -24.3293) ccw projected
  line L5 (-21.0542, -17.0685) -> (-24.5794, -15.8528) projected
  line L6 (-24.5794, -15.8528) -> (-18.8508, 0.7585) projected
  arc A7 (-2.9036, 6.9168) -> (-18.8508, 0.7585) centre (0, -24.3293) ccw projected
  line L7 (-2.9036, 6.9168) -> (-4.7386, 1.596) projected
  line L8 (-4.7386, 1.596) -> (-4.7384, 1.596) projected
  spline S0 degree 7 poles (-4.7386, 1.596) (-4.7646, 1.5189) (-4.789, 1.4413) (-4.812, 1.3634) (-4.8335, 1.2851) (-4.8535, 1.2065) (-4.872, 1.1276) (-4.9552, 0.7394) (-4.9987, 0.4257) (-5.0192, 0.1077) (-5.0163, -0.2137) (-4.9891, -0.5378) (-4.9364, -0.8636) (-4.8108, -1.376) (-4.7564, -1.5622) (-4.6928, -1.7483) (-4.6197, -1.934) (-4.5366, -2.119) (-4.4432, -2.3028) (-4.3388, -2.485) knots 0 0 0 0 0 0 0 0 0.14045 0.14045 0.14045 0.14045 0.14045 0.14045 0.687772 0.687772 0.687772 0.687772 0.687772 0.687772 1 1 1 1 1 1 1 1 projected
  arc A8 (4.3388, -2.485) -> (-4.3388, -2.485) centre (0, -24.3293) ccw projected
  spline S1 degree 7 poles (4.3388, -2.4849) (4.4051, -2.3691) (4.4671, -2.2526) (4.5247, -2.1356) (4.5782, -2.0181) (4.6277, -1.9003) (4.6732, -1.7823) (4.7149, -1.6641) knots 0 0 0 0 0 0 0 0 1 1 1 1 1 1 1 1 projected
  line L9 (4.7149, -1.6641) -> (4.7151, -1.6642) projected
  line L10 (-2.9036, 6.9168) -> (-1.622, 10.6331)
  arc A9 (8.599, 9.598) -> (-1.622, 10.6331) centre (0, -24.3293) ccw projected
  line L11 (8.599, 9.598) -> (7.4144, 6.163)
  point P0 (-4.3388, -2.485)
  point P1 (4.3388, -2.485)
  dimension "d342" = 5
  dimension "d316" = 5
  dimension "d317" = 5
  constraints: 4 end point, 1 point on circle, 2 other
  measures "d342" distance from line of L10 A0.centre
extrude "押し出し66" cut sketch "スケッチ60" against normal blind 11.5
